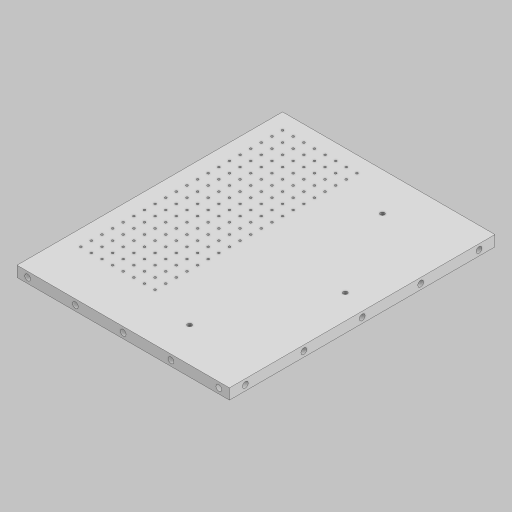
# Autodesk Inventor part: podstawa_baza
Saved by Autodesk Inventor 2024.3 (Build 283343000, 343)
## iProperties
Created: 2025-10-10
Part Number: podstawa_baza
Material: Ogólny
Document SubType Name: Modeling
Designer: User
Density: 1 g/cm^3
Appearance: Domyślna
Mass: 490.94 g
Surface Area: 1154.28 cm^2
Volume: 490.94 cm^3
Author: User
Autodesk Inventor part; units mm, degrees
ref_plane "YZ Plane" through (0, 0, 0) normal (1, 0, 0) x (0, 1, 0)
sketch "Szkic1" plane through (0, 0, 0) normal (0, 1, 0) x (-1, 0, 0)
  line L0 (0, 0) -> (200, 0)
  line L1 (200, 0) -> (200, -250)
  line L2 (200, -250) -> (0, -250)
  line L3 (0, -250) -> (0, 0)
  line L4 (0, 0) -> (0, -15)
  line L5 (0, -15) -> (15, -15)
  line L6 (15, -15) -> (75, -15)
  line L7 (75, -15) -> (75, -235)
  line L8 (75, -235) -> (15, -235)
  line L9 (15, -235) -> (15, -15)
  line L10 (200, -250) -> (185, -250)
  line L11 (185, -250) -> (185, -235)
  line L12 (185, -235) -> (115, -235)
  line L13 (115, -235) -> (115, -145)
  line L14 (115, -145) -> (185, -145)
  line L15 (185, -145) -> (185, -235)
  line L16 (100, -250) -> (100, -170)
  circle A0 centre (100, -170) radius 15
  line L17 (100, -170) -> (100, -106.66)
  circle A1 centre (100, -106.66) radius 11
  line L18 (79, -85.66) -> (121, -85.66)
  line L19 (121, -85.66) -> (121, -127.66)
  line L20 (121, -127.66) -> (79, -127.66)
  line L21 (79, -127.66) -> (79, -85.66)
  line L22 (79, -85.66) -> (121, -127.66) construction
  line L23 (121, -85.66) -> (79, -127.66) construction
  line L24 (75, -15) -> (15, -235)
  line L25 (75, -235) -> (15, -15)
  circle A2 centre (45, -125) radius 10.1096
  line L26 (15, -9.1027) -> (15, -235)
  line L27 (15, -235) -> (15, -15)
  line L28 (15, -15) -> (75, -15)
  line L29 (75, -15) -> (75, -235)
  line L30 (75, -235) -> (15, -235)
  line L31 (75, -15) -> (75, -32.5)
  line L32 (75, -32.5) -> (70, -32.5)
  circle A3 centre (70, -32.5) radius 2
  line L33 (75, -235) -> (75, -214)
  line L34 (75, -214) -> (70, -214)
  circle A4 centre (70, -214) radius 2
  line L35 (15, -15) -> (23, -15)
  line L36 (23, -15) -> (23, -132)
  circle A5 centre (23, -132) radius 2
  point P0 (7, 7.17)
  dimension "d0" = 200
  dimension "d1" = 250
  dimension "d2" = 15
  dimension "d3" = 15
  dimension "d4" = 60
  dimension "d5" = 220
  dimension "d6" = 15
  dimension "d7" = 15
  dimension "d8" = 70
  dimension "d9" = 90
  dimension "d10" = 80
  dimension "d11" = 30
  dimension "d12" = 63.34
  dimension "d13" = 22
  dimension "d14" = 42
  dimension "d15" = 42
  dimension "d51" = 220
  dimension "d52" = 60
  dimension "d53" = 17.5
  dimension "d54" = 5
  dimension "d55" = 4
  dimension "d56" = 21
  dimension "d57" = 5
  dimension "d58" = 4
  dimension "d59" = 8
  dimension "d60" = 117
  dimension "d61" = 4
  constraints: 74 end point, 11 parallel, 9 perpendicular, 6 centre point, 5 coincident, 5 point on line, 4 horizontal, 4 midpoint, 2 vertical
  measures "d0" distance of L1.end L2.end
  measures "d1" distance of L0.end L1.end
  measures "d2" distance of L0.start L4.end
  measures "d3" distance of L4.end L5.end
  measures "d4" distance of L7.end L8.end
  measures "d5" distance of L6.end L7.end
  measures "d6" distance of L1.end L10.end
  measures "d7" distance of L10.end L11.end
  measures "d8" distance of L13.end L14.end
  measures "d9" distance of L12.end L13.end
  measures "d10" distance of L16.start L16.end
  measures "d11" diameter of A0
  measures "d12" distance of L17.start L17.end
  measures "d13" diameter of A1
  measures "d14" distance of L19.end L20.end
  measures "d15" distance of L18.end L19.end
  measures "d51" distance of L29.start L33.start
  measures "d52" distance of L27.end L29.start
  measures "d53" distance of L29.start L32.start
  measures "d54" distance of L32.start L32.end
  measures "d55" diameter of A3
  measures "d56" distance of L33.start L34.start
  measures "d57" distance of L34.start L34.end
  measures "d58" diameter of A4
  measures "d59" distance of L27.end L36.start
  measures "d60" distance of L36.start L36.end
  measures "d61" diameter of A5
extrude "Wyciągnięcie proste1" add sketch "Szkic1" along normal blind 10 contours L6 L36 L25 | A5 | L25 A2 L24 L9 | A1 | L20 L21 L18 L19 | L0 L1 L2 L11 L15 L14 L13 A0 L16 L3 | L2 L16 A0 L13 L12 L11 | L6 L24 A3 A2 L25 L36 | L24 A2 L25 A4 L8 | L12 L13 L14 L15 | A0 L17 L16 | L16 L17 A0 | L7 L32 A3 L24 | L25 A4 L34 L7 | A2 L25 L24 | L24 L25 A2 | A2 L24 L25 | L7 L34 A4 L25 A2 L24 A3 L32 | A3 L32 L24 | L24 A3 | A4 L25 | L25 A4 | L24 A2 L25 | A3 L24 L32
sketch "Szkic2" plane through (0, 0, 0) normal (1, 0, 0) x (0, 0, -1)
  line L0 (0, 0) -> (0, 10) projected
  line L1 (0, 5) -> (15, 5)
  circle A0 centre (15, 5) radius 2.75
  line L2 (250, 0) -> (250, 10) projected
  line L3 (250, 5) -> (235, 5)
  circle A1 centre (70, 5) radius 2.75
  circle A2 centre (125, 5) radius 2.75
  circle A3 centre (180, 5) radius 2.75
  circle A4 centre (235, 5) radius 2.75
  dimension "d18" = 15
  dimension "d19" = 5.5
  dimension "d20" = 15
  dimension "d46" = 55
  constraints: 5 centre point, 4 end point, 3 horizontal, 2 midpoint, 1 coincident, 8 other
  measures "d18" distance of L1.start L1.end
  measures "d19" diameter of A0
  measures "d20" distance of L3.start L3.end
  measures "d46" distance of A0.centre A1.centre
sketch "Szkic3" plane through (-200, 0, 0) normal (0, 0, 1) x (1, 0, 0)
  line L0 (0, 0) -> (0, 10) projected
  line L1 (0, 5) -> (10, 5)
  line L2 (200, 5) -> (190, 5)
  circle A0 centre (10, 5) radius 2.75
  circle A1 centre (55, 5) radius 2.75
  circle A2 centre (100, 5) radius 2.75
  circle A3 centre (145, 5) radius 2.75
  circle A4 centre (190, 5) radius 2.75
  point P0 (200, 0)
  dimension "d28" = 10
  dimension "d29" = 10
  dimension "d30" = 5.5
  dimension "d36" = 45
  constraints: 5 centre point, 4 end point, 3 horizontal, 1 coincident, 1 midpoint, 8 other
  measures "d28" distance of L1.start L1.end
  measures "d29" distance of L2.start L2.end
  measures "d30" diameter of A0
  measures "d36" distance of A0.centre A1.centre
ref_plane "Płaszczyzna konstrukcyjna1" through (-100, 0, 0) normal (1, 0, 0) x (0, 0, -1)
ref_plane "Płaszczyzna konstrukcyjna2" through (-200, 0, -125) normal (0, 0, 1) x (1, 0, 0)
extrude "Wyciągnięcie proste2" cut sketch "Szkic3" against normal blind 20
extrude "Wyciągnięcie proste3" cut sketch "Szkic2" against normal blind 20
mirror "Odbij1" about plane through (-100, 0, 0) normal (1, 0, 0) of "Wyciągnięcie proste3"
mirror "Odbij2" about plane through (-200, 0, -125) normal (0, 0, 1) of "Wyciągnięcie proste2"
extrude "Wyciągnięcie proste4" cut sketch "Szkic1" along normal blind 45 contours A5 | A3 L32 L24 | L24 A3 | A4 L25 | L25 A4 | A3 L24 L32
sketch "Szkic4" plane through (0, 10, 0) normal (0, 1, 0) x (1, 0, 0)
  line L0 (-200, 250) -> (-200, 0) projected
  line L1 (-200, 250) -> (-185, 250)
  line L2 (0, 250) -> (-200, 250) projected
  line L3 (-185, 250) -> (-185, 235)
  circle A0 centre (-185, 235) radius 1
  circle A1 centre (-185, 225) radius 1
  circle A2 centre (-185, 215) radius 1
  circle A3 centre (-185, 205) radius 1
  circle A4 centre (-185, 195) radius 1
  circle A5 centre (-185, 185) radius 1
  circle A6 centre (-185, 175) radius 1
  circle A7 centre (-185, 165) radius 1
  circle A8 centre (-185, 155) radius 1
  circle A9 centre (-185, 145) radius 1
  circle A10 centre (-185, 135) radius 1
  circle A11 centre (-185, 125) radius 1
  circle A12 centre (-185, 115) radius 1
  circle A13 centre (-185, 105) radius 1
  circle A14 centre (-185, 95) radius 1
  circle A15 centre (-185, 85) radius 1
  circle A16 centre (-185, 75) radius 1
  circle A17 centre (-185, 65) radius 1
  circle A18 centre (-185, 55) radius 1
  circle A19 centre (-185, 45) radius 1
  circle A20 centre (-175, 235) radius 1
  circle A21 centre (-175, 225) radius 1
  circle A22 centre (-175, 215) radius 1
  circle A23 centre (-175, 205) radius 1
  circle A24 centre (-175, 195) radius 1
  circle A25 centre (-175, 185) radius 1
  circle A26 centre (-175, 175) radius 1
  circle A27 centre (-175, 165) radius 1
  circle A28 centre (-175, 155) radius 1
  circle A29 centre (-175, 145) radius 1
  circle A30 centre (-175, 135) radius 1
  circle A31 centre (-175, 125) radius 1
  circle A32 centre (-175, 115) radius 1
  circle A33 centre (-175, 105) radius 1
  circle A34 centre (-175, 95) radius 1
  circle A35 centre (-175, 85) radius 1
  circle A36 centre (-175, 75) radius 1
  circle A37 centre (-175, 65) radius 1
  circle A38 centre (-175, 55) radius 1
  circle A39 centre (-175, 45) radius 1
  circle A40 centre (-165, 235) radius 1
  circle A41 centre (-165, 225) radius 1
  circle A42 centre (-165, 215) radius 1
  circle A43 centre (-165, 205) radius 1
  circle A44 centre (-165, 195) radius 1
  circle A45 centre (-165, 185) radius 1
  circle A46 centre (-165, 175) radius 1
  circle A47 centre (-165, 165) radius 1
  circle A48 centre (-165, 155) radius 1
  circle A49 centre (-165, 145) radius 1
  circle A50 centre (-165, 135) radius 1
  circle A51 centre (-165, 125) radius 1
  circle A52 centre (-165, 115) radius 1
  circle A53 centre (-165, 105) radius 1
  circle A54 centre (-165, 95) radius 1
  circle A55 centre (-165, 85) radius 1
  circle A56 centre (-165, 75) radius 1
  circle A57 centre (-165, 65) radius 1
  circle A58 centre (-165, 55) radius 1
  circle A59 centre (-165, 45) radius 1
  circle A60 centre (-155, 235) radius 1
  circle A61 centre (-155, 225) radius 1
  circle A62 centre (-155, 215) radius 1
  circle A63 centre (-155, 205) radius 1
  circle A64 centre (-155, 195) radius 1
  circle A65 centre (-155, 185) radius 1
  circle A66 centre (-155, 175) radius 1
  circle A67 centre (-155, 165) radius 1
  circle A68 centre (-155, 155) radius 1
  circle A69 centre (-155, 145) radius 1
  circle A70 centre (-155, 135) radius 1
  circle A71 centre (-155, 125) radius 1
  circle A72 centre (-155, 115) radius 1
  circle A73 centre (-155, 105) radius 1
  circle A74 centre (-155, 95) radius 1
  circle A75 centre (-155, 85) radius 1
  circle A76 centre (-155, 75) radius 1
  circle A77 centre (-155, 65) radius 1
  circle A78 centre (-155, 55) radius 1
  circle A79 centre (-155, 45) radius 1
  circle A80 centre (-145, 235) radius 1
  circle A81 centre (-145, 225) radius 1
  circle A82 centre (-145, 215) radius 1
  circle A83 centre (-145, 205) radius 1
  circle A84 centre (-145, 195) radius 1
  circle A85 centre (-145, 185) radius 1
  circle A86 centre (-145, 175) radius 1
  circle A87 centre (-145, 165) radius 1
  circle A88 centre (-145, 155) radius 1
  circle A89 centre (-145, 145) radius 1
  circle A90 centre (-145, 135) radius 1
  circle A91 centre (-145, 125) radius 1
  circle A92 centre (-145, 115) radius 1
  circle A93 centre (-145, 105) radius 1
  circle A94 centre (-145, 95) radius 1
  circle A95 centre (-145, 85) radius 1
  circle A96 centre (-145, 75) radius 1
  circle A97 centre (-145, 65) radius 1
  circle A98 centre (-145, 55) radius 1
  circle A99 centre (-145, 45) radius 1
  circle A100 centre (-135, 235) radius 1
  circle A101 centre (-135, 225) radius 1
  circle A102 centre (-135, 215) radius 1
  circle A103 centre (-135, 205) radius 1
  circle A104 centre (-135, 195) radius 1
  circle A105 centre (-135, 185) radius 1
  circle A106 centre (-135, 175) radius 1
  circle A107 centre (-135, 165) radius 1
  circle A108 centre (-135, 155) radius 1
  circle A109 centre (-135, 145) radius 1
  circle A110 centre (-135, 135) radius 1
  circle A111 centre (-135, 125) radius 1
  circle A112 centre (-135, 115) radius 1
  circle A113 centre (-135, 105) radius 1
  circle A114 centre (-135, 95) radius 1
  circle A115 centre (-135, 85) radius 1
  circle A116 centre (-135, 75) radius 1
  circle A117 centre (-135, 65) radius 1
  circle A118 centre (-135, 55) radius 1
  circle A119 centre (-135, 45) radius 1
  circle A120 centre (-125, 235) radius 1
  circle A121 centre (-125, 225) radius 1
  circle A122 centre (-125, 215) radius 1
  circle A123 centre (-125, 205) radius 1
  circle A124 centre (-125, 195) radius 1
  circle A125 centre (-125, 185) radius 1
  circle A126 centre (-125, 175) radius 1
  circle A127 centre (-125, 165) radius 1
  circle A128 centre (-125, 155) radius 1
  circle A129 centre (-125, 145) radius 1
  circle A130 centre (-125, 135) radius 1
  circle A131 centre (-125, 125) radius 1
  circle A132 centre (-125, 115) radius 1
  circle A133 centre (-125, 105) radius 1
  circle A134 centre (-125, 95) radius 1
  circle A135 centre (-125, 85) radius 1
  circle A136 centre (-125, 75) radius 1
  circle A137 centre (-125, 65) radius 1
  circle A138 centre (-125, 55) radius 1
  circle A139 centre (-125, 45) radius 1
  circle A140 centre (-115, 235) radius 1
  circle A141 centre (-115, 225) radius 1
  circle A142 centre (-115, 215) radius 1
  circle A143 centre (-115, 205) radius 1
  circle A144 centre (-115, 195) radius 1
  circle A145 centre (-115, 185) radius 1
  circle A146 centre (-115, 175) radius 1
  circle A147 centre (-115, 165) radius 1
  circle A148 centre (-115, 155) radius 1
  circle A149 centre (-115, 145) radius 1
  circle A150 centre (-115, 135) radius 1
  circle A151 centre (-115, 125) radius 1
  circle A152 centre (-115, 115) radius 1
  circle A153 centre (-115, 105) radius 1
  circle A154 centre (-115, 95) radius 1
  circle A155 centre (-115, 85) radius 1
  circle A156 centre (-115, 75) radius 1
  circle A157 centre (-115, 65) radius 1
  circle A158 centre (-115, 55) radius 1
  circle A159 centre (-115, 45) radius 1
  point P0 (0, 0)
  dimension "d64" = 15
  dimension "d65" = 15
  dimension "d66" = 2
  dimension "d69" = 10
  dimension "d72" = 10
  constraints: 160 centre point, 4 end point, 1 coincident, 1 horizontal, 1 perpendicular, 1 point on line, 1 vertical, 318 other
  measures "d64" distance of L0.start L1.end
  measures "d65" distance of L1.end L3.end
  measures "d66" diameter of A0
  measures "d69" distance of A0.centre A1.centre
  measures "d72" distance of A0.centre A20.centre
extrude "Wyciągnięcie proste5" cut sketch "Szkic4" against normal blind 45
sketch "Szkic5" plane through (0, 0, 0) normal (0, -1, 0) x (1, 0, 0)
  line L0 (0, -250) -> (-200, -250) projected
  line L1 (-200, -250) -> (-185, -250)
  line L2 (-185, -250) -> (-185, -235)
  circle A0 centre (-185, -235) radius 2
  circle A1 centre (-185, -225) radius 2
  circle A2 centre (-185, -215) radius 2
  circle A3 centre (-185, -205) radius 2
  circle A4 centre (-185, -195) radius 2
  circle A5 centre (-185, -185) radius 2
  circle A6 centre (-185, -175) radius 2
  circle A7 centre (-185, -165) radius 2
  circle A8 centre (-185, -155) radius 2
  circle A9 centre (-185, -145) radius 2
  circle A10 centre (-185, -135) radius 2
  circle A11 centre (-185, -125) radius 2
  circle A12 centre (-185, -115) radius 2
  circle A13 centre (-185, -105) radius 2
  circle A14 centre (-185, -95) radius 2
  circle A15 centre (-185, -85) radius 2
  circle A16 centre (-185, -75) radius 2
  circle A17 centre (-185, -65) radius 2
  circle A18 centre (-185, -55) radius 2
  circle A19 centre (-185, -45) radius 2
  circle A20 centre (-175, -235) radius 2
  circle A21 centre (-175, -225) radius 2
  circle A22 centre (-175, -215) radius 2
  circle A23 centre (-175, -205) radius 2
  circle A24 centre (-175, -195) radius 2
  circle A25 centre (-175, -185) radius 2
  circle A26 centre (-175, -175) radius 2
  circle A27 centre (-175, -165) radius 2
  circle A28 centre (-175, -155) radius 2
  circle A29 centre (-175, -145) radius 2
  circle A30 centre (-175, -135) radius 2
  circle A31 centre (-175, -125) radius 2
  circle A32 centre (-175, -115) radius 2
  circle A33 centre (-175, -105) radius 2
  circle A34 centre (-175, -95) radius 2
  circle A35 centre (-175, -85) radius 2
  circle A36 centre (-175, -75) radius 2
  circle A37 centre (-175, -65) radius 2
  circle A38 centre (-175, -55) radius 2
  circle A39 centre (-175, -45) radius 2
  circle A40 centre (-165, -235) radius 2
  circle A41 centre (-165, -225) radius 2
  circle A42 centre (-165, -215) radius 2
  circle A43 centre (-165, -205) radius 2
  circle A44 centre (-165, -195) radius 2
  circle A45 centre (-165, -185) radius 2
  circle A46 centre (-165, -175) radius 2
  circle A47 centre (-165, -165) radius 2
  circle A48 centre (-165, -155) radius 2
  circle A49 centre (-165, -145) radius 2
  circle A50 centre (-165, -135) radius 2
  circle A51 centre (-165, -125) radius 2
  circle A52 centre (-165, -115) radius 2
  circle A53 centre (-165, -105) radius 2
  circle A54 centre (-165, -95) radius 2
  circle A55 centre (-165, -85) radius 2
  circle A56 centre (-165, -75) radius 2
  circle A57 centre (-165, -65) radius 2
  circle A58 centre (-165, -55) radius 2
  circle A59 centre (-165, -45) radius 2
  circle A60 centre (-155, -235) radius 2
  circle A61 centre (-155, -225) radius 2
  circle A62 centre (-155, -215) radius 2
  circle A63 centre (-155, -205) radius 2
  circle A64 centre (-155, -195) radius 2
  circle A65 centre (-155, -185) radius 2
  circle A66 centre (-155, -175) radius 2
  circle A67 centre (-155, -165) radius 2
  circle A68 centre (-155, -155) radius 2
  circle A69 centre (-155, -145) radius 2
  circle A70 centre (-155, -135) radius 2
  circle A71 centre (-155, -125) radius 2
  circle A72 centre (-155, -115) radius 2
  circle A73 centre (-155, -105) radius 2
  circle A74 centre (-155, -95) radius 2
  circle A75 centre (-155, -85) radius 2
  circle A76 centre (-155, -75) radius 2
  circle A77 centre (-155, -65) radius 2
  circle A78 centre (-155, -55) radius 2
  circle A79 centre (-155, -45) radius 2
  circle A80 centre (-145, -235) radius 2
  circle A81 centre (-145, -225) radius 2
  circle A82 centre (-145, -215) radius 2
  circle A83 centre (-145, -205) radius 2
  circle A84 centre (-145, -195) radius 2
  circle A85 centre (-145, -185) radius 2
  circle A86 centre (-145, -175) radius 2
  circle A87 centre (-145, -165) radius 2
  circle A88 centre (-145, -155) radius 2
  circle A89 centre (-145, -145) radius 2
  circle A90 centre (-145, -135) radius 2
  circle A91 centre (-145, -125) radius 2
  circle A92 centre (-145, -115) radius 2
  circle A93 centre (-145, -105) radius 2
  circle A94 centre (-145, -95) radius 2
  circle A95 centre (-145, -85) radius 2
  circle A96 centre (-145, -75) radius 2
  circle A97 centre (-145, -65) radius 2
  circle A98 centre (-145, -55) radius 2
  circle A99 centre (-145, -45) radius 2
  circle A100 centre (-135, -235) radius 2
  circle A101 centre (-135, -225) radius 2
  circle A102 centre (-135, -215) radius 2
  circle A103 centre (-135, -205) radius 2
  circle A104 centre (-135, -195) radius 2
  circle A105 centre (-135, -185) radius 2
  circle A106 centre (-135, -175) radius 2
  circle A107 centre (-135, -165) radius 2
  circle A108 centre (-135, -155) radius 2
  circle A109 centre (-135, -145) radius 2
  circle A110 centre (-135, -135) radius 2
  circle A111 centre (-135, -125) radius 2
  circle A112 centre (-135, -115) radius 2
  circle A113 centre (-135, -105) radius 2
  circle A114 centre (-135, -95) radius 2
  circle A115 centre (-135, -85) radius 2
  circle A116 centre (-135, -75) radius 2
  circle A117 centre (-135, -65) radius 2
  circle A118 centre (-135, -55) radius 2
  circle A119 centre (-135, -45) radius 2
  circle A120 centre (-125, -235) radius 2
  circle A121 centre (-125, -225) radius 2
  circle A122 centre (-125, -215) radius 2
  circle A123 centre (-125, -205) radius 2
  circle A124 centre (-125, -195) radius 2
  circle A125 centre (-125, -185) radius 2
  circle A126 centre (-125, -175) radius 2
  circle A127 centre (-125, -165) radius 2
  circle A128 centre (-125, -155) radius 2
  circle A129 centre (-125, -145) radius 2
  circle A130 centre (-125, -135) radius 2
  circle A131 centre (-125, -125) radius 2
  circle A132 centre (-125, -115) radius 2
  circle A133 centre (-125, -105) radius 2
  circle A134 centre (-125, -95) radius 2
  circle A135 centre (-125, -85) radius 2
  circle A136 centre (-125, -75) radius 2
  circle A137 centre (-125, -65) radius 2
  circle A138 centre (-125, -55) radius 2
  circle A139 centre (-125, -45) radius 2
  circle A140 centre (-115, -235) radius 2
  circle A141 centre (-115, -225) radius 2
  circle A142 centre (-115, -215) radius 2
  circle A143 centre (-115, -205) radius 2
  circle A144 centre (-115, -195) radius 2
  circle A145 centre (-115, -185) radius 2
  circle A146 centre (-115, -175) radius 2
  circle A147 centre (-115, -165) radius 2
  circle A148 centre (-115, -155) radius 2
  circle A149 centre (-115, -145) radius 2
  circle A150 centre (-115, -135) radius 2
  circle A151 centre (-115, -125) radius 2
  circle A152 centre (-115, -115) radius 2
  circle A153 centre (-115, -105) radius 2
  circle A154 centre (-115, -95) radius 2
  circle A155 centre (-115, -85) radius 2
  circle A156 centre (-115, -75) radius 2
  circle A157 centre (-115, -65) radius 2
  circle A158 centre (-115, -55) radius 2
  circle A159 centre (-115, -45) radius 2
  point P0 (0, 0)
  dimension "d77" = 15
  dimension "d78" = 15
  dimension "d79" = 90
  dimension "d80" = 4
  dimension "d83" = 10
  dimension "d86" = 10
  constraints: 160 centre point, 4 end point, 1 coincident, 1 horizontal, 1 perpendicular, 1 point on line, 1 vertical, 318 other
  measures "d77" distance of L0.end L1.end
  measures "d78" distance of L1.end L2.end
  measures "d79" angle of L2 L1
  measures "d80" diameter of A0
  measures "d83" distance of A0.centre A1.centre
  measures "d86" distance of A0.centre A20.centre
extrude "Wyciągnięcie proste6" cut sketch "Szkic5" against normal blind 1
